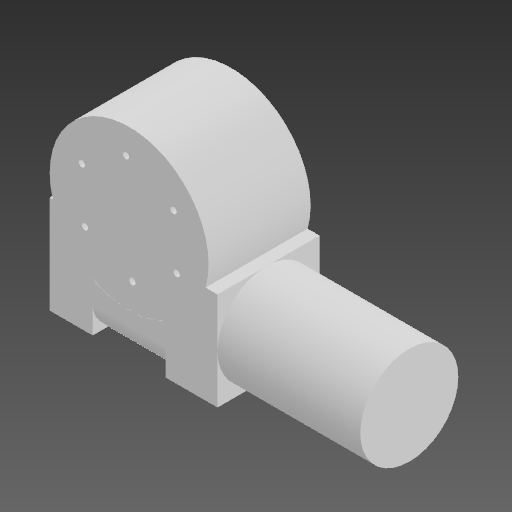
# Autodesk Inventor part: RotaryPlatform
Saved by Autodesk Inventor 2020 (Build 240168000, 168)
## iProperties
Created: 2020-05-14
Part Number: RotaryPlatform
Material: Generic
Document SubType Name: Modeling
Designer: valer
Density: 1 g/cm^3
Appearance: Default
Author: valer
Autodesk Inventor part; units mm, degrees
ref_plane "YZ Plane" through (0, 0, 0) normal (1, 0, 0) x (0, 1, 0)
ref_plane "XZ Plane" through (0, 0, 0) normal (0, 1, 0) x (-1, 0, 0)
ref_plane "XY Plane" through (0, 0, 0) normal (0, 0, 1) x (1, 0, 0)
sketch "Sketch3" plane through (0, 0, 0) normal (0, 0, 1) x (1, 0, 0)
  circle A0 centre (0, 0) radius 76
  circle A1 centre (0, 0) radius 12.7
  circle A2 centre (0, 0) radius 50.8
  circle A3 centre (-45.4162, 22.7599) radius 3
  circle A4 centre (0, 12.7) radius 3
  line L0 (-76, 0) -> (76, 0)
  line L1 (76, 0) -> (76, -114.3)
  line L2 (76, -114.3) -> (-76, -114.3)
  line L3 (-76, -114.3) -> (-76, 0)
  circle A5 centre (-42.4187, -27.9516) radius 3
  circle A6 centre (2.9974, -50.7115) radius 3
  circle A7 centre (45.4162, -22.7599) radius 3
  circle A8 centre (42.4187, 27.9516) radius 3
  circle A9 centre (-2.9974, 50.7115) radius 3
  circle A10 centre (-12.7, 0) radius 3
  circle A11 centre (0, -12.7) radius 3
  circle A12 centre (12.7, 0) radius 3
  line L4 (-76, -20.6375) -> (-34.925, -20.6375)
  line L5 (-34.925, -20.6375) -> (-34.925, -114.3)
  line L6 (-34.925, -114.3) -> (-76, -114.3)
  line L7 (-76, -114.3) -> (-76, -20.6375)
  line L8 (0, 0) -> (0, -114.3) construction
  line L9 (76, -20.6375) -> (34.925, -20.6375)
  line L10 (34.925, -20.6375) -> (34.925, -114.3)
  line L11 (-2.9974, 50.7115) -> (-2.9974, 0) construction
  point P0 (34.925, -67.5)
  point P1 (73.1443, -20.6375)
  point P2 (-34.925, -67.5)
  dimension "d5" = 152
  dimension "d20" = 101.6
  dimension "d21" = 25.4
  dimension "d8" = 6
  dimension "d9" = 6
  dimension "d12" = 360
  dimension "d16" = 360
  dimension "d22" = 114.3
  constraints: 24 end point, 10 centre point, 5 point on line, 4 parallel, 3 coincident, 3 perpendicular, 3 symmetric about line, 2 horizontal, 1 midpoint, 1 vertical, 1 vertical alignment, 30 other
  measures "d8" diameter of A3
  measures "d9" diameter of A4
  measures "d22" distance of L0.end L1.end
extrude "Extrusion3" add sketch "Sketch3" along normal mid plane 97.5 contours L0 A2 A8 A9 A3 A0 | A0 L9 A7 A2 L0 | L0 A2 L4 A0 | A0 L10 A2 A7 L9 | L0 A12 A1 A4 A10 A2 A3 A9 A8 | A2 A7 L9 L10 A6 L5 L4 L0 A10 A1 A11 A12 | L4 A2 A5 L5 A0 | A0 L5 A2 A6 L10 | L9 A2 A7 | A7 A2 L9 | A8 A2 | A2 A8 | A2 L9 A7 | A12 A1 L0 | L0 A1 A12 | L4 L5 A2 A5 | A3 A2 | A2 A3 | A10 A1 L0 | L0 A1 A10 | L10 L9 A7 A2 | A2 A7 L9 | L0 A12 A1 | A1 A12 L0 | A12 L0 A10 A1 A4 | A1 A11 A10 L0 A12 | A5 A2 | A2 A5 | L0 A10 A1 | A1 A10 L0 | A6 A2 | A2 A6 | A9 A2 | A2 A9 | A4 A1 | A1 A4 | A11 A1 | A1 A11
extrude "Extrusion4" add sketch "Sketch3" along normal mid plane 97.5 contours L9 L1 L2 L10 A0 | L4 A2 A5 L5 A0 | A0 L5 L2 L3 L4 | L4 L5 A2 A5 | A5 A2 | A2 A5
extrude "Extrusion5" add sketch "Sketch3" along normal mid plane 97.5 separate body contours L10 L2 L5 A0
fillet "Fillet1" radius 25.4 2 edges at (0, -114.3, 48.75) (0, -114.3, -48.75)
sketch "Sketch4" plane through (76, -114.3, 48.75) normal (1, 0, 0) x (0, 0, -1)
  line L0 (0, 0) -> (0, 93.6625) projected
  line L1 (97.5, 0) -> (0, 0) projected
  line L2 (97.5, 93.6625) -> (97.5, 0) projected
  line L3 (97.5, 0) -> (0, 0) projected
  line L4 (97.5, 0) -> (97.5, 93.6625) projected
  line L5 (0, 0) -> (97.5, 0)
  line L6 (97.5, 0) -> (97.5, 93.6625)
  line L7 (97.5, 93.6625) -> (0, 93.6625)
  line L8 (0, 93.6625) -> (0, 0)
  point P0 (48.75, 114.3)
  constraints: 8 end point, 2 parallel, 1 horizontal, 1 perpendicular
extrude "Extrusion6" add sketch "Sketch4" along normal blind 8.4667 bodies 1
sketch "Sketch5" plane through (84.4667, -114.3, 48.75) normal (1, 0, 0) x (0, 0, -1)
  line L0 (0, 93.6625) -> (0, 0) projected
  line L1 (0, 0) -> (97.5, 0) projected
  line L2 (97.5, 0) -> (97.5, 93.6625) projected
  line L3 (97.5, 93.6625) -> (0, 93.6625) projected
  line L4 (0, 93.6625) -> (0, 0) projected
  circle A0 centre (46.8313, 46.8313) radius 46.8313
  line L5 (97.5, 93.6625) -> (0, 93.6625) projected
  line L6 (0, 0) -> (97.5, 0) projected
  point P0 (48.75, 114.3)
  constraints: 3 tangent, 1 centre point
extrude "Extrusion7" add sketch "Sketch5" along normal blind 136.652 contours A0 bodies 1
sketch "Sketch6" plane through (0, 0, 48.75) normal (0, 0, 1) x (1, 0, 0)
  circle A0 centre (-45.4162, 22.7599) radius 3 projected
  circle A1 centre (-2.9974, 50.7115) radius 3 projected
  circle A2 centre (42.4187, 27.9516) radius 3 projected
  circle A3 centre (45.4162, -22.7599) radius 3 projected
  circle A4 centre (2.9974, -50.7115) radius 3 projected
  circle A5 centre (-42.4187, -27.9516) radius 3 projected
  point P0 (0, 0)
hole "Hole1" at (-42.4187, -27.9516, 48.75) at (-45.4162, 22.7599, 48.75) at (-2.9974, 50.7115, 48.75) at (42.4187, 27.9516, 48.75) at (45.4162, -22.7599, 48.75) at (2.9974, -50.7115, 48.75) direction (0, 0, -1) diameter 6 end through all bodies 1
body "Solid2"
body "Solid3"
